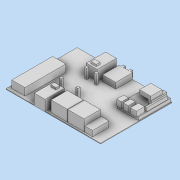
# Autodesk Inventor part: body
Saved by Autodesk Inventor 2022 (Build 260153000, 153)
## iProperties
Created: 2022-09-24
Part Number: body
Material: Générique
Document SubType Name: Modeling
Designer: andre
Density: 1 g/cm^3
Appearance: Par défaut
Author: andre
Autodesk Inventor part; units mm, degrees
ref_plane "YZ Plane" through (0, 0, 0) normal (1, 0, 0) x (0, 1, 0)
ref_plane "XZ Plane" through (0, 0, 0) normal (0, 1, 0) x (-1, 0, 0)
ref_plane "XY Plane" through (0, 0, 0) normal (0, 0, 1) x (1, 0, 0)
sketch "Esquisse1" plane through (0, 0, 0) normal (0, 1, 0) x (-1, 0, 0)
  line L0 (125.5, 94.5) -> (-125.5, 94.5)
  line L1 (-125.5, 94.5) -> (-125.5, -94.5)
  line L2 (-125.5, -94.5) -> (125.5, -94.5)
  line L3 (125.5, -94.5) -> (125.5, 94.5)
  line L4 (125.5, 94.5) -> (-125.5, -94.5) construction
  line L5 (-125.5, 94.5) -> (125.5, -94.5) construction
  point P0 (0, 0)
  dimension "d0" = 251
  dimension "d1" = 189
  constraints: 12 end point, 2 midpoint, 2 parallel, 1 horizontal, 1 perpendicular
  measures "d0" distance of L0.start L0.end
  measures "d1" distance of L2.end L0.start
extrude "Extrusion1" add sketch "Esquisse1" along normal blind 1.8
sketch "Esquisse2" plane through (0, 1.8, 0) normal (0, 1, 0) x (1, 0, 0)
  line L0 (124, 93) -> (67.9, 93)
  line L1 (67.9, 93) -> (67.9, 7.5)
  line L2 (67.9, 7.5) -> (124, 7.5)
  line L3 (124, 7.5) -> (124, 93)
  line L4 (125.5, 94.5) -> (-125.5, 94.5) projected
  line L5 (125.5, -94.5) -> (125.5, 94.5) projected
  point P0 (0, 0)
  dimension "d4" = 1.5
  dimension "d5" = 1.5
  dimension "d6" = 56.1
  dimension "d7" = 85.5
  constraints: 8 end point, 2 parallel, 1 horizontal, 1 perpendicular
  measures "d4" distance between parallel lines of L4 L0
  measures "d5" distance between parallel lines of L5 L3
  measures "d6" distance of L1.end L2.end
  measures "d7" distance of L0.end L1.end
extrude "Extrusion2" add sketch "Esquisse2" along normal blind 8.7
sketch "Esquisse3" plane through (0, 10.5, 0) normal (0, 1, 0) x (1, 0, 0)
  line L0 (121.8, 25.8) -> (105.8, 25.8)
  line L1 (105.8, 25.8) -> (105.8, 4.4)
  line L2 (105.8, 4.4) -> (121.8, 4.4)
  line L3 (121.8, 4.4) -> (121.8, 25.8)
  line L4 (124, 7.5) -> (124, 93) projected
  line L5 (67.9, 7.5) -> (124, 7.5) projected
  point P0 (0, 0)
  dimension "d10" = 21.4
  dimension "d11" = 16
  dimension "d12" = 2.2
  dimension "d13" = 3.1
  constraints: 8 end point, 2 parallel, 1 horizontal, 1 perpendicular
  measures "d10" distance of L2.end L0.start
  measures "d11" distance of L1.end L2.end
  measures "d12" distance between parallel lines of L4 L3
  measures "d13" distance between parallel lines of L5 L2
extrude "Extrusion3" add sketch "Esquisse3" along normal blind 13.5
sketch "Esquisse4" plane through (0, 10.5, 0) normal (0, 1, 0) x (1, 0, 0)
  line L0 (69.9, 22.7) -> (83, 22.7)
  line L1 (83, 22.7) -> (83, 4.4)
  line L2 (83, 4.4) -> (69.9, 4.4)
  line L3 (69.9, 4.4) -> (69.9, 22.7)
  line L4 (67.9, 93) -> (67.9, 7.5) projected
  line L5 (105.8, 4.4) -> (121.8, 4.4) projected
  line L6 (87.5, 4.4) -> (100.6, 4.4)
  line L7 (100.6, 4.4) -> (100.6, 22.7)
  line L8 (100.6, 22.7) -> (87.5, 22.7)
  line L9 (87.5, 22.7) -> (87.5, 4.4)
  point P0 (0, 0)
  point P1 (76.45, 4.4)
  point P2 (76.45, 22.7)
  dimension "d16" = 13.1
  dimension "d17" = 18.3
  dimension "d18" = 2
  dimension "d19" = 4.5
  dimension "d20" = 13.1
  constraints: 16 end point, 4 parallel, 3 point on line, 2 horizontal, 2 midpoint, 2 perpendicular
  measures "d16" distance of L1.end L2.end
  measures "d17" distance of L2.end L0.start
  measures "d18" distance between parallel lines of L3 L4
  measures "d19" distance between parallel lines of L1 L9
  measures "d20" distance of L6.start L6.end
extrude "Extrusion4" add sketch "Esquisse4" along normal blind 15.5
sketch "Esquisse5" plane through (0, 10.5, 0) normal (0, 1, 0) x (1, 0, 0)
  line L0 (123, 86) -> (118.5, 86)
  line L1 (118.5, 86) -> (118.5, 29.6)
  line L2 (118.5, 29.6) -> (123, 29.6)
  line L3 (123, 29.6) -> (123, 86)
  line L4 (124, 7.5) -> (124, 93) projected
  line L5 (124, 93) -> (67.9, 93) projected
  point P0 (0, 0)
  dimension "d23" = 56.4
  dimension "d24" = 4.5
  dimension "d25" = 1
  dimension "d26" = 7
  constraints: 8 end point, 2 parallel, 1 horizontal, 1 perpendicular
  measures "d23" distance of L0.end L1.end
  measures "d24" distance of L0.start L0.end
  measures "d25" distance between parallel lines of L4 L3
  measures "d26" distance between parallel lines of L5 L0
extrude "Extrusion5" add sketch "Esquisse5" along normal blind 9
sketch "Esquisse6" plane through (0, 10.5, 0) normal (0, 1, 0) x (1, 0, 0)
  line L0 (118.5, 29.6) -> (118.5, 86) projected
  line L1 (118.5, 86) -> (118.5, 88.7)
  line L2 (118.5, 88.7) -> (109.5, 88.7)
  line L3 (109.5, 88.7) -> (109.5, 47.7)
  line L4 (109.5, 47.7) -> (118.5, 47.7)
  line L5 (124, 93) -> (67.9, 93) projected
  point P0 (0, 0)
  dimension "d29" = 9
  dimension "d30" = 41
  dimension "d31" = 4.3
  constraints: 8 end point, 3 perpendicular, 1 point on line, 1 vertical
  measures "d29" distance between parallel lines of L0 L3
  measures "d30" distance of L2.end L3.end
  measures "d31" distance between parallel lines of L5 L2
extrude "Extrusion6" add sketch "Esquisse6" along normal blind 13.6
sketch "Esquisse7" plane through (0, 24.1, 0) normal (0, 1, 0) x (1, 0, 0)
  line L0 (118.5, 47.7) -> (109.5, 47.7) projected
  line L1 (116.8, 47.7) -> (86.8, 47.7)
  line L2 (86.8, 47.7) -> (86.8, 77.7)
  line L3 (86.8, 77.7) -> (116.8, 77.7)
  line L4 (116.8, 77.7) -> (116.8, 47.7)
  line L5 (118.5, 47.7) -> (118.5, 88.7) projected
  point P0 (0, 0)
  dimension "d34" = 30
  dimension "d35" = 30
  dimension "d36" = 1.7
  constraints: 8 end point, 2 parallel, 1 horizontal, 1 perpendicular, 1 point on line
  measures "d34" distance of L1.start L1.end
  measures "d35" distance of L1.end L2.end
  measures "d36" distance between parallel lines of L5 L4
extrude "Extrusion7" add sketch "Esquisse7" along normal blind 10.3
sketch "Esquisse8" plane through (0, 1.8, 0) normal (0, 1, 0) x (1, 0, 0)
  line L0 (125.5, 94.5) -> (-125.5, 94.5) projected
  line L1 (-50.4, 94.5) -> (-21.3, 94.5)
  line L2 (-21.3, 94.5) -> (-21.3, 43.5)
  line L3 (-21.3, 43.5) -> (-50.4, 43.5)
  line L4 (-50.4, 43.5) -> (-50.4, 94.5)
  line L5 (-125.5, 94.5) -> (-125.5, -94.5) projected
  point P0 (0, 0)
  dimension "d39" = 75.1
  dimension "d40" = 29.1
  dimension "d41" = 51
  constraints: 8 end point, 2 parallel, 1 horizontal, 1 perpendicular, 1 point on line
  measures "d39" distance between parallel lines of L5 L4
  measures "d40" distance between parallel lines of L2 L4
  measures "d41" distance of L3.end L1.start
extrude "Extrusion8" add sketch "Esquisse8" along normal blind 27.3
sketch "Esquisse9" plane through (0, 29.1, 0) normal (0, 1, 0) x (1, 0, 0)
  line L0 (-28.85, 48.5) -> (-42.85, 48.5)
  line L1 (-42.85, 48.5) -> (-42.85, 58.5)
  line L2 (-42.85, 58.5) -> (-28.85, 58.5)
  line L3 (-28.85, 58.5) -> (-28.85, 48.5)
  line L4 (-21.3, 43.5) -> (-21.3, 94.5) projected
  line L5 (-50.4, 94.5) -> (-50.4, 43.5) projected
  line L6 (-21.3, 94.5) -> (-50.4, 94.5) projected
  point P0 (0, 0)
  dimension "d44" = 10
  dimension "d45" = 14
  dimension "d46" = 7.55
  dimension "d47" = 7.55
  dimension "d48" = 36
  constraints: 8 end point, 2 parallel, 1 horizontal, 1 perpendicular
  measures "d44" distance of L0.end L1.end
  measures "d45" distance of L0.start L0.end
  measures "d46" distance between parallel lines of L3 L4
  measures "d47" distance between parallel lines of L5 L1
  measures "d48" distance between parallel lines of L2 L6
extrude "Extrusion9" add sketch "Esquisse9" along normal blind 5
mirror "Symétrie1" about plane through (0, 0, 0) normal (0, 0, 1) of "Extrusion8", "Extrusion9"
sketch "Esquisse10" plane through (0, 1.8, 0) normal (0, 1, 0) x (1, 0, 0)
  line L0 (125.5, 94.5) -> (-21.3, 94.5) projected
  line L1 (-13.8, 94.5) -> (21.4, 94.5)
  line L2 (21.4, 94.5) -> (21.4, 50)
  line L3 (21.4, 50) -> (-13.8, 50)
  line L4 (-13.8, 50) -> (-13.8, 94.5)
  line L5 (16.4, 94.5) -> (10.4, 94.5)
  line L6 (10.4, 94.5) -> (10.4, 100.5)
  line L7 (10.4, 100.5) -> (16.4, 100.5)
  line L8 (16.4, 100.5) -> (16.4, 94.5)
  line L9 (-2.8, 94.5) -> (-8.8, 94.5)
  line L10 (-8.8, 94.5) -> (-8.8, 100.5)
  line L11 (-8.8, 100.5) -> (-2.8, 100.5)
  line L12 (-2.8, 100.5) -> (-2.8, 94.5)
  line L13 (-21.3, 43.5) -> (-21.3, 94.5) projected
  point P0 (0, 0)
  point P1 (21.4, 94.5)
  point P2 (-2.8, 94.5)
  point P3 (-8.8, 94.5)
  dimension "d51" = 44.5
  dimension "d52" = 35.2
  dimension "d53" = 6
  dimension "d54" = 6
  dimension "d55" = 6
  dimension "d56" = 5
  dimension "d57" = 5
  dimension "d115" = 7.5
  constraints: 24 end point, 6 parallel, 4 point on line, 3 horizontal, 3 perpendicular
  measures "d51" distance of L1.end L2.end
  measures "d52" distance of L2.end L3.end
  measures "d53" distance of L6.end L7.end
  measures "d54" distance of L10.end L11.end
  measures "d55" distance of L7.end L5.start
  measures "d56" distance between parallel lines of L2 L8
  measures "d57" distance between parallel lines of L4 L10
  measures "d115" distance between parallel lines of L13 L4
extrude "Extrusion10" add sketch "Esquisse10" along normal blind 15.5
sketch "Esquisse11" plane through (0, 1.8, 0) normal (0, 1, 0) x (1, 0, 0)
  line L0 (-9.8, -90.5) -> (33.3, -90.5)
  line L1 (33.3, -90.5) -> (33.3, -47.4)
  line L2 (33.3, -47.4) -> (-9.8, -47.4)
  line L3 (-9.8, -47.4) -> (-9.8, -90.5)
  line L4 (34.8, -90.5) -> (77.9, -90.5)
  line L5 (77.9, -90.5) -> (77.9, -47.4)
  line L6 (77.9, -47.4) -> (34.8, -47.4)
  line L7 (34.8, -47.4) -> (34.8, -90.5)
  line L8 (-21.3, -94.5) -> (125.5, -94.5) projected
  line L9 (-21.3, -43.5) -> (-21.3, -94.5) projected
  point P0 (0, 0)
  dimension "d60" = 43.1
  dimension "d61" = 43.1
  dimension "d62" = 43.1
  dimension "d63" = 4
  dimension "d64" = 1.5
  dimension "d65" = 11.5
  constraints: 16 end point, 4 parallel, 2 horizontal, 2 perpendicular, 2 point on line
  measures "d60" distance of L0.start L0.end
  measures "d61" distance of L0.end L1.end
  measures "d62" distance of L4.start L4.end
  measures "d63" distance between parallel lines of L8 L0
  measures "d64" distance between parallel lines of L1 L7
  measures "d65" distance between parallel lines of L9 L3
extrude "Extrusion11" add sketch "Esquisse11" along normal blind 30
sketch "Esquisse12" plane through (0, 1.8, 0) normal (0, 1, 0) x (1, 0, 0)
  line L0 (-117.8, -86.9) -> (-82.8, -86.9)
  line L1 (-82.8, -86.9) -> (-82.8, 21.6)
  line L2 (-82.8, 21.6) -> (-117.8, 21.6)
  line L3 (-117.8, 21.6) -> (-117.8, -86.9)
  line L4 (-125.5, -94.5) -> (-50.4, -94.5) projected
  line L5 (-125.5, 94.5) -> (-125.5, -94.5) projected
  point P0 (0, 0)
  dimension "d68" = 108.5
  dimension "d69" = 35
  dimension "d70" = 7.6
  dimension "d71" = 7.7
  constraints: 8 end point, 2 parallel, 1 horizontal, 1 perpendicular
  measures "d68" distance of L2.end L0.start
  measures "d69" distance of L0.start L0.end
  measures "d70" distance between parallel lines of L4 L0
  measures "d71" distance between parallel lines of L5 L3
extrude "Extrusion12" add sketch "Esquisse12" along normal blind 20
sketch "Esquisse13" plane through (0, 1.8, 0) normal (0, 1, 0) x (1, 0, 0)
  line L0 (-21.3, -43.5) -> (-21.3, -94.5) projected
  line L1 (-4, -25) -> (-10, -25)
  line L2 (-10, -25) -> (-10, -19)
  line L3 (-10, -19) -> (-4, -19)
  line L4 (-4, -19) -> (-4, -25)
  line L5 (-4, -25) -> (-10, -19) construction
  line L6 (-10, -25) -> (-4, -19) construction
  line L7 (-48, -25) -> (-54, -25)
  line L8 (-54, -25) -> (-54, -19)
  line L9 (-54, -19) -> (-48, -19)
  line L10 (-48, -19) -> (-48, -25)
  line L11 (-48, -25) -> (-54, -19) construction
  line L12 (-54, -25) -> (-48, -19) construction
  line L13 (-7, -22) -> (-51, -22)
  line L14 (-125.5, -94.5) -> (-50.4, -94.5) projected
  line L15 (-125.5, 94.5) -> (-125.5, -94.5) projected
  line L16 (-39, 33) -> (-45, 33)
  line L17 (-45, 33) -> (-45, 39)
  line L18 (-45, 39) -> (-39, 39)
  line L19 (-39, 39) -> (-39, 33)
  line L20 (-39, 33) -> (-45, 39) construction
  line L21 (-45, 33) -> (-39, 39) construction
  line L22 (-42, 36) -> (-16, 36)
  line L23 (-13, 33) -> (-19, 33)
  line L24 (-19, 33) -> (-19, 39)
  line L25 (-19, 39) -> (-13, 39)
  line L26 (-13, 39) -> (-13, 33)
  line L27 (-13, 33) -> (-19, 39) construction
  line L28 (-19, 33) -> (-13, 39) construction
  point P0 (0, 0)
  dimension "d87" = 6
  dimension "d88" = 6
  dimension "d89" = 6
  dimension "d90" = 6
  dimension "d91" = 72.5
  dimension "d92" = 74.5
  dimension "d93" = 44
  dimension "d94" = 6
  dimension "d95" = 6
  dimension "d96" = 6
  dimension "d97" = 6
  dimension "d98" = 58
  dimension "d99" = 9
  dimension "d101" = 26
  dimension "d102" = 9
  constraints: 52 end point, 8 midpoint, 8 parallel, 6 horizontal, 4 perpendicular
  measures "d87" distance of L1.end L2.end
  measures "d88" distance of L1.start L1.end
  measures "d89" distance of L7.start L7.end
  measures "d90" distance of L7.end L8.end
  measures "d91" distance between parallel lines of L14 L13
  measures "d92" distance from line of L15 L13.end
  measures "d93" distance of L13.end L13.start
  measures "d94" distance of L16.end L17.end
  measures "d95" distance of L16.start L16.end
  measures "d96" distance of L23.start L23.end
  measures "d97" distance of L25.end L23.start
  measures "d98" distance between parallel lines of L13 L22
  measures "d99" horizontal distance of L13.start L22.end
  measures "d101" distance of L22.start L22.end
  measures "d102" horizontal distance of L22.start L13.end
extrude "Extrusion13" add sketch "Esquisse13" along normal blind 26
sketch "Esquisse14" plane through (0, 0, 0) normal (0, 0, 1) x (1, 0, 0)
  line L0 (125.5, 0) -> (-125.5, 0) projected
  line L1 (76, 0) -> (76, -7.4346)
  line L2 (68.5, 0) -> (68.5, -9.1)
  arc A0 (68.5, -9.1) -> (76, -7.4346) centre (68.5, 8.6202) ccw
  line L3 (125.5, 0) -> (125.5, 1.8) projected
  point P0 (0, 0)
  dimension "d105" = 9.1
  dimension "d106" = 7.5
  dimension "d107" = 49.5
  constraints: 4 end point, 2 point on circle, 2 point on line, 1 centre point, 1 line through centre, 1 perpendicular, 1 vertical
  measures "d105" distance of L2.start L2.end
  measures "d106" distance between parallel lines of L2 L1
  measures "d107" distance between parallel lines of L3 L1
revolve "Révolution1" add sketch "Esquisse14" angle 360 about axis through (68.5, 0, 0) along (0, -1, 0)
sketch "Esquisse15" plane through (0, 1.8, 0) normal (0, 1, 0) x (1, 0, 0)
  line L0 (79.6, -90.5) -> (100.5, -90.5)
  line L1 (100.5, -90.5) -> (100.5, -47.3)
  line L2 (100.5, -47.3) -> (79.6, -47.3)
  line L3 (79.6, -47.3) -> (79.6, -90.5)
  line L4 (-21.3, -94.5) -> (125.5, -94.5) projected
  line L5 (34.8, -90.5) -> (77.9, -90.5) projected
  line L6 (77.9, -90.5) -> (77.9, -47.4) projected
  point P0 (0, 0)
  dimension "d109" = 20.9
  dimension "d110" = 43.2
  dimension "d112" = 1.7
  constraints: 8 end point, 2 parallel, 1 horizontal, 1 perpendicular, 1 point on line
  measures "d109" distance of L0.start L0.end
  measures "d110" distance of L0.end L1.end
  measures "d112" distance between parallel lines of L6 L3
extrude "Extrusion14" add sketch "Esquisse15" along normal blind 14.8
equation "\"d5\" = d4"
equation "\"d20\" = d16"
equation "\"d35\" = d34"
equation "\"d46\" = d47"
equation "\"d54\" = d53"
equation "\"d55\" = d53"
equation "\"d57\" = d56"
equation "\"d61\" = d60"
equation "\"d62\" = d60"
equation "\"d88\" = d87"
equation "\"d89\" = d88"
equation "\"d90\" = d87"
equation "\"d94\" = d88"
equation "\"d95\" = d94"
equation "\"d96\" = d95"
equation "\"d97\" = d94"
equation "\"d99\" = d102"
